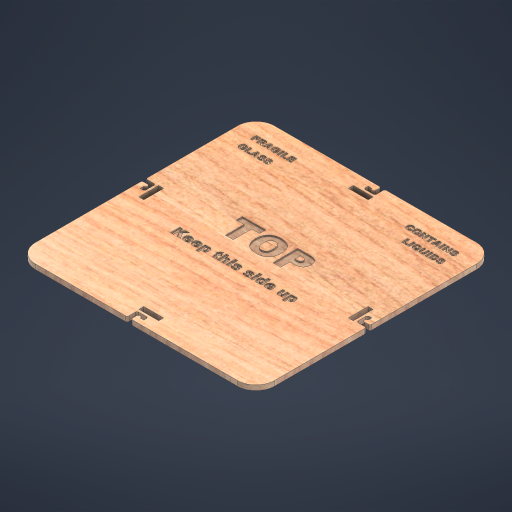
# Autodesk Inventor part: Lid
Saved by Autodesk Inventor 2024.1 (Build 281209000, 209)
## iProperties
Created: 2024-05-23
Part Number: Lid
Material: Wood (Birch)
Document SubType Name: Modeling
Designer: Tim Jäger
Density: 0.55 g/cm^3
Appearance: Birch - Natural Polished
Author: Tim Jäger
Autodesk Inventor part; units mm, degrees
(part 1 of 2)
ref_plane "YZ Plane" through (0, 0, 0) normal (1, 0, 0) x (0, 1, 0)
ref_plane "XZ Plane" through (0, 0, 0) normal (0, 1, 0) x (-1, 0, 0)
ref_plane "XY Plane" through (0, 0, 0) normal (0, 0, 1) x (1, 0, 0)
sketch "Sketch1" plane through (0, 0, 0) normal (0, 1, 0) x (-1, 0, 0)
  line L0 (-82, 97) -> (82, 97)
  line L1 (97, 82) -> (97, -82)
  line L2 (82, -97) -> (-82, -97)
  line L3 (-97, -82) -> (-97, 82)
  line L4 (-97, 97) -> (97, -97) construction
  line L5 (97, 97) -> (-97, -97) construction
  arc A0 (82, -97) -> (97, -82) centre (82, -82) ccw
  arc A1 (-97, -82) -> (-82, -97) centre (-82, -82) ccw
  arc A2 (-82, 97) -> (-97, 82) centre (-82, 82) ccw
  arc A3 (97, 82) -> (82, 97) centre (82, 82) ccw
  line L6 (97, -7.5) -> (89, -7.5)
  line L7 (89, -7.5) -> (89, 1.5)
  line L8 (89, 1.5) -> (91, 1.5)
  line L9 (91, 1.5) -> (91, -1.5) construction
  line L10 (91, -4.5) -> (97, -4.5)
  line L11 (91, 1.5) -> (92.5, 1.5)
  line L12 (92.5, 1.5) -> (92.5, -1.5)
  line L13 (92.5, -1.5) -> (91, -1.5)
  line L14 (91, -1.5) -> (91, 1.5) construction
  line L15 (91, -1.5) -> (91, -4.5)
  line L16 (-1.5, 89) -> (-1.5, 91)
  line L17 (-1.5, 91) -> (-1.5, 92.5)
  line L18 (-1.5, 91) -> (1.5, 91) construction
  line L19 (1.5, 91) -> (-1.5, 91) construction
  line L20 (-1.5, 92.5) -> (1.5, 92.5)
  line L21 (1.5, 91) -> (4.5, 91)
  line L22 (7.5, 89) -> (-1.5, 89)
  line L23 (4.5, 91) -> (4.5, 97)
  line L24 (7.5, 97) -> (7.5, 89)
  line L25 (1.5, 92.5) -> (1.5, 91)
  line L26 (-89, -1.5) -> (-91, -1.5)
  line L27 (-91, -1.5) -> (-92.5, -1.5)
  line L28 (-91, -1.5) -> (-91, 1.5) construction
  line L29 (-91, 1.5) -> (-91, -1.5) construction
  line L30 (-92.5, -1.5) -> (-92.5, 1.5)
  line L31 (-91, 1.5) -> (-91, 4.5)
  line L32 (-89, 7.5) -> (-89, -1.5)
  line L33 (-91, 4.5) -> (-97, 4.5)
  line L34 (-97, 7.5) -> (-89, 7.5)
  line L35 (-92.5, 1.5) -> (-91, 1.5)
  line L36 (1.5, -89) -> (1.5, -91)
  line L37 (1.5, -91) -> (1.5, -92.5)
  line L38 (1.5, -91) -> (-1.5, -91) construction
  line L39 (-1.5, -91) -> (1.5, -91) construction
  line L40 (1.5, -92.5) -> (-1.5, -92.5)
  line L41 (-1.5, -91) -> (-4.5, -91)
  line L42 (-7.5, -89) -> (1.5, -89)
  line L43 (-4.5, -91) -> (-4.5, -97)
  line L44 (-7.5, -97) -> (-7.5, -89)
  line L45 (-1.5, -92.5) -> (-1.5, -91)
  line L46 (8, -87) -> (-8, -87)
  line L47 (-8, -87) -> (-8, -83)
  line L48 (-8, -83) -> (8, -83)
  line L49 (8, -83) -> (8, -87)
  line L50 (87, -8) -> (83, -8)
  line L51 (83, -8) -> (83, 8)
  line L52 (83, 8) -> (87, 8)
  line L53 (87, 8) -> (87, -8)
  line L54 (8, 87) -> (8, 83)
  line L55 (8, 83) -> (-8, 83)
  line L56 (-8, 83) -> (-8, 87)
  line L57 (-8, 87) -> (8, 87)
  line L58 (-87, 8) -> (-83, 8)
  line L59 (-83, 8) -> (-83, -8)
  line L60 (-83, -8) -> (-87, -8)
  line L61 (-87, -8) -> (-87, 8)
  point P0 (0, 0)
  point P1 (93, -7.5)
  point P2 (92.5, 0)
  point P3 (0, 92.5)
  point P4 (7.5, 93)
  point P5 (-92.5, 0)
  point P6 (-93, 7.5)
  point P7 (0, -92.5)
  point P8 (-7.5, -93)
  point P9 (7.5, 97)
  point P10 (4.5, 97)
  point P11 (-97, 7.5)
  point P12 (-97, 4.5)
  point P13 (-7.5, -97)
  point P14 (-4.5, -97)
  point P15 (0, -87)
  point P16 (0, -83)
  point P17 (83, 0)
  point P18 (87, 0)
  point P19 (0, 0)
  point P20 (0, 83)
  point P21 (0, 87)
  point P22 (0, 0)
  point P23 (-83, 0)
  point P24 (-87, 0)
  point P25 (0, 0)
  dimension "d16" = 15
  dimension "d17" = 6
  dimension "d18" = 3
  dimension "d19" = 6
  dimension "d20" = 3
  dimension "d21" = 1.5
  dimension "d24" = 360
  dimension "d29" = 4
  dimension "d30" = 16
  dimension "d31" = 83
  dimension "d32" = 2
  dimension "d33" = 194
  dimension "d34" = 194
  dimension "d37" = 360
  constraints: 124 end point, 10 point on line, 8 perpendicular, 8 point on circle, 8 tangent, 6 midpoint, 6 parallel, 4 centre point, 4 horizontal, 3 equal radius, 2 coincident, 1 horizontal alignment, 1 vertical alignment, 128 other
  measures "d16" radius of A0
  measures "d17" distance between parallel lines of L1 L9
  measures "d18" distance from line of point (93, -7.5) L10
  measures "d19" distance of L8.end L10.start
  measures "d20" distance of L11.end L12.end
  measures "d21" distance of L12.end L9.end
  measures "d29" distance of L46.end L47.end
  measures "d30" distance of L46.start L46.end
  measures "d31" distance of point (0, 0) point (0, -83)
  measures "d32" distance between parallel lines of L7 L15
  measures "d33" distance between parallel lines of L1 L3
  measures "d34" distance between parallel lines of L0 L2
extrude "Extrusion1" add sketch "Sketch1" along normal blind 4 contours L0 L23 L21 L25 L20 L17 L16 L22 L24 A3 L1 L10 L15 L13 L12 L11 L8 L7 L6 A0 L2 L43 L41 L45 L40 L37 L36 L42 L44 A1 L3 L33 L31 L35 L30 L27 L26 L32 L34 A2
fillet "Fillet1" radius 1.5 24 edges at (-4.5, 2, 97) (-7.5, 2, 97) (-7.5, 2, 89) (-4.5, 2, 91) (1.5, 2, 89) (-1.5, 2, 91) (89, 2, 7.5) (97, 2, 7.5) (97, 2, 4.5) (91, 2, 4.5) (91, 2, 1.5) (89, 2, -1.5) (-1.5, 2, -89) (1.5, 2, -91) (4.5, 2, -91) (7.5, 2, -89) (4.5, 2, -97) (7.5, 2, -97) (-97, 2, -4.5) (-97, 2, -7.5) (-91, 2, -4.5) (-91, 2, -1.5) (-89, 2, 1.5) (-89, 2, -7.5)
sketch "Sketch2" plane through (0, 4, 0) normal (0, 1, 0) x (1, 0, 0)
  line L0 (-37.5, 25) -> (37.5, 25) construction
  line L1 (37.5, 25) -> (37.5, -5) construction
  line L2 (37.5, -5) -> (-37.5, -5) construction
  line L3 (-37.5, -5) -> (-37.5, 25) construction
  line L4 (-65, -10) -> (65, -10) construction
  line L5 (65, -10) -> (65, -25) construction
  line L6 (65, -25) -> (-65, -25) construction
  line L7 (-65, -25) -> (-65, -10) construction
  line L8 (0, 25) -> (0, -25) construction
  line L9 (-31.2031, 20.1697) -> (-12.3965, 20.1697)
  line L10 (-12.3965, 20.1697) -> (-12.3965, 15.2226)
  line L11 (-12.3965, 15.2226) -> (-18.7103, 15.2226)
  line L12 (-18.7103, 15.2226) -> (-18.7103, 0.1697)
  line L13 (-18.7103, 0.1697) -> (-24.8893, 0.1697)
  line L14 (-24.8893, 0.1697) -> (-24.8893, 15.2226)
  line L15 (-24.8893, 15.2226) -> (-31.2031, 15.2226)
  line L16 (-31.2031, 15.2226) -> (-31.2031, 20.1697)
  spline S0 degree 2 poles (-10.3754, 10.16) (-10.3754, 15.0493) (-4.9086, 20.5161) (-0.0385, 20.5161) knots 0 0 0 1 2 2 2
  spline S1 degree 2 poles (-0.0385, 20.5161) (4.9471, 20.5161) (10.3561, 15.1456) (10.3561, 10.314) knots 0 0 0 1 2 2 2
  spline S2 degree 2 poles (10.3561, 10.314) (10.3561, 6.8107) (7.9885, 2.3256) (3.5226, -0.1768) (0.1925, -0.1768) knots 0 0 0 1 2 3 3 3
  spline S3 degree 2 poles (0.1925, -0.1768) (-3.1761, -0.1768) (-7.6227, 1.9791) (-10.3754, 6.6567) (-10.3754, 10.16) knots 0 0 0 1 2 3 3 3
  spline S4 degree 2 poles (-4.1963, 10.1215) (-4.1963, 7.0994) (-1.9442, 4.443) (0, 4.443) knots 0 0 0 1 2 2 2
  spline S5 degree 2 poles (0, 4.443) (1.9827, 4.443) (4.1771, 7.0416) (4.1771, 10.391) knots 0 0 0 1 2 2 2
  spline S6 degree 2 poles (4.1771, 10.391) (4.1771, 13.2207) (1.9057, 15.8386) (-0.0577, 15.8386) knots 0 0 0 1 2 2 2
  spline S7 degree 2 poles (-0.0577, 15.8386) (-1.9249, 15.8386) (-4.1963, 13.1822) (-4.1963, 10.1215) knots 0 0 0 1 2 2 2
  line L17 (13.667, 20.1697) -> (23.9461, 20.1697)
  spline S8 degree 2 poles (23.9461, 20.1697) (27.2955, 20.1697) (30.6449, 16.9743) (30.6449, 14.0291) knots 0 0 0 1 2 2 2
  spline S9 degree 2 poles (30.6449, 14.0291) (30.6449, 10.9878) (27.0067, 7.5806) (23.2724, 7.5806) knots 0 0 0 1 2 2 2
  line L18 (23.2724, 7.5806) -> (19.8845, 7.5806)
  line L19 (19.8845, 7.5806) -> (19.8845, 0.1697)
  line L20 (19.8845, 0.1697) -> (13.667, 0.1697)
  line L21 (13.667, 0.1697) -> (13.667, 20.1697)
  line L22 (19.8845, 11.6422) -> (21.3859, 11.6422)
  spline S10 degree 2 poles (21.3859, 11.6422) (23.1761, 11.6422) (24.6198, 12.8934) (24.6198, 13.8559) knots 0 0 0 1 2 2 2
  spline S11 degree 2 poles (24.6198, 13.8559) (24.6198, 14.7991) (23.3686, 16.1081) (21.6362, 16.1081) knots 0 0 0 1 2 2 2
  line L23 (21.6362, 16.1081) -> (19.8845, 16.1081)
  line L24 (19.8845, 16.1081) -> (19.8845, 11.6422)
  line L25 (-49.0315, -12.7178) -> (-46.7144, -12.7178)
  line L26 (-46.7144, -12.7178) -> (-46.7144, -15.5546)
  line L27 (-46.7144, -15.5546) -> (-44.2818, -12.7178)
  line L28 (-44.2818, -12.7178) -> (-41.1995, -12.7178)
  line L29 (-41.1995, -12.7178) -> (-43.9353, -15.5474)
  line L30 (-43.9353, -15.5474) -> (-41.0768, -20.2178)
  line L31 (-41.0768, -20.2178) -> (-43.9353, -20.2178)
  line L32 (-43.9353, -20.2178) -> (-45.5161, -17.1355)
  line L33 (-45.5161, -17.1355) -> (-46.7144, -18.3987)
  line L34 (-46.7144, -18.3987) -> (-46.7144, -20.2178)
  line L35 (-46.7144, -20.2178) -> (-49.0315, -20.2178)
  line L36 (-49.0315, -20.2178) -> (-49.0315, -12.7178)
  line L37 (-34.4141, -18.0161) -> (-38.5864, -18.0161)
  spline S12 degree 2 poles (-38.5864, -18.0161) (-38.5286, -18.5214) (-38.3121, -18.7668) knots 0 0 0 1 1 1
  spline S13 degree 2 poles (-38.3121, -18.7668) (-38.0161, -19.1205) (-37.5253, -19.1205) knots 0 0 0 1 1 1
  spline S14 degree 2 poles (-37.5253, -19.1205) (-37.2221, -19.1205) (-36.9406, -18.969) knots 0 0 0 1 1 1
  spline S15 degree 2 poles (-36.9406, -18.969) (-36.7745, -18.8679) (-36.5796, -18.6225) knots 0 0 0 1 1 1
  line L38 (-36.5796, -18.6225) -> (-34.5296, -18.8102)
  spline S16 degree 2 poles (-34.5296, -18.8102) (-34.9988, -19.6258) (-36.3342, -20.3405) (-37.5758, -20.3405) knots 0 0 0 1 2 2 2
  spline S17 degree 2 poles (-37.5758, -20.3405) (-38.6586, -20.3405) (-39.8929, -19.7341) (-40.7086, -18.4059) (-40.7086, -17.5108) knots 0 0 0 1 2 3 3 3
  spline S18 degree 2 poles (-40.7086, -17.5108) (-40.7086, -16.2332) (-39.0772, -14.6595) (-37.6408, -14.6595) knots 0 0 0 1 2 2 2
  spline S19 degree 2 poles (-37.6408, -14.6595) (-36.4714, -14.6595) (-35.1215, -15.3669) (-34.4141, -16.7096) (-34.4141, -17.7779) knots 0 0 0 1 2 3 3 3
  line L39 (-34.4141, -17.7779) -> (-34.4141, -18.0161)
  spline S20 degree 2 poles (-36.5363, -17.02) (-36.5941, -16.4136) (-37.121, -15.8939) (-37.5541, -15.8939) knots 0 0 0 1 2 2 2
  spline S21 degree 2 poles (-37.5541, -15.8939) (-38.045, -15.8939) (-38.341, -16.2909) knots 0 0 0 1 1 1
  spline S22 degree 2 poles (-38.341, -16.2909) (-38.5286, -16.5363) (-38.5792, -17.02) knots 0 0 0 1 1 1
  line L40 (-38.5792, -17.02) -> (-36.5363, -17.02)
  line L41 (-27.4194, -18.0161) -> (-31.5917, -18.0161)
  spline S23 degree 2 poles (-31.5917, -18.0161) (-31.5339, -18.5214) (-31.3174, -18.7668) knots 0 0 0 1 1 1
  spline S24 degree 2 poles (-31.3174, -18.7668) (-31.0214, -19.1205) (-30.5306, -19.1205) knots 0 0 0 1 1 1
  spline S25 degree 2 poles (-30.5306, -19.1205) (-30.2274, -19.1205) (-29.9459, -18.969) knots 0 0 0 1 1 1
  spline S26 degree 2 poles (-29.9459, -18.969) (-29.7798, -18.8679) (-29.5849, -18.6225) knots 0 0 0 1 1 1
  line L42 (-29.5849, -18.6225) -> (-27.5349, -18.8102)
  spline S27 degree 2 poles (-27.5349, -18.8102) (-28.0041, -19.6258) (-29.3395, -20.3405) (-30.5811, -20.3405) knots 0 0 0 1 2 2 2
  spline S28 degree 2 poles (-30.5811, -20.3405) (-31.6639, -20.3405) (-32.8982, -19.7341) (-33.7139, -18.4059) (-33.7139, -17.5108) knots 0 0 0 1 2 3 3 3
  spline S29 degree 2 poles (-33.7139, -17.5108) (-33.7139, -16.2332) (-32.0825, -14.6595) (-30.6461, -14.6595) knots 0 0 0 1 2 2 2
  spline S30 degree 2 poles (-30.6461, -14.6595) (-29.4767, -14.6595) (-28.1268, -15.3669) (-27.4194, -16.7096) (-27.4194, -17.7779) knots 0 0 0 1 2 3 3 3
  line L43 (-27.4194, -17.7779) -> (-27.4194, -18.0161)
  spline S31 degree 2 poles (-29.5416, -17.02) (-29.5994, -16.4136) (-30.1263, -15.8939) (-30.5594, -15.8939) knots 0 0 0 1 2 2 2
  spline S32 degree 2 poles (-30.5594, -15.8939) (-31.0503, -15.8939) (-31.3462, -16.2909) knots 0 0 0 1 1 1
  spline S33 degree 2 poles (-31.3462, -16.2909) (-31.5339, -16.5363) (-31.5845, -17.02) knots 0 0 0 1 1 1
  line L44 (-31.5845, -17.02) -> (-29.5416, -17.02)
  line L45 (-26.4449, -22.2822) -> (-26.4449, -14.7822)
  line L46 (-26.4449, -14.7822) -> (-24.4959, -14.7822)
  line L47 (-24.4959, -14.7822) -> (-24.4959, -15.5835)
  spline S34 degree 2 poles (-24.4959, -15.5835) (-24.0917, -15.0782) (-23.7596, -14.8977) knots 0 0 0 1 1 1
  spline S35 degree 2 poles (-23.7596, -14.8977) (-23.2976, -14.6595) (-22.749, -14.6595) knots 0 0 0 1 1 1
  spline S36 degree 2 poles (-22.749, -14.6595) (-21.659, -14.6595) (-20.468, -16.327) (-20.468, -17.5541) knots 0 0 0 1 2 2 2
  spline S37 degree 2 poles (-20.468, -17.5541) (-20.468, -18.9112) (-21.7673, -20.3405) (-22.7563, -20.3405) knots 0 0 0 1 2 2 2
  spline S38 degree 2 poles (-22.7563, -20.3405) (-23.2399, -20.3405) (-24.0339, -20.0156) (-24.3443, -19.6908) knots 0 0 0 1 2 2 2
  line L48 (-24.3443, -19.6908) -> (-24.3443, -22.2822)
  line L49 (-24.3443, -22.2822) -> (-26.4449, -22.2822)
  spline S39 degree 2 poles (-24.3588, -17.5108) (-24.3588, -18.1605) (-23.8174, -18.7813) (-23.4059, -18.7813) knots 0 0 0 1 2 2 2
  spline S40 degree 2 poles (-23.4059, -18.7813) (-23.045, -18.7813) (-22.5541, -18.1821) (-22.5541, -17.4675) knots 0 0 0 1 2 2 2
  spline S41 degree 2 poles (-22.5541, -17.4675) (-22.5541, -16.8106) (-23.0666, -16.1898) (-23.4348, -16.1898) knots 0 0 0 1 2 2 2
  spline S42 degree 2 poles (-23.4348, -16.1898) (-23.8318, -16.1898) (-24.3588, -16.8106) (-24.3588, -17.5108) knots 0 0 0 1 2 2 2
  line L50 (-13.4589, -12.7178) -> (-13.4589, -14.7822)
  line L51 (-13.4589, -14.7822) -> (-12.3111, -14.7822)
  line L52 (-12.3111, -14.7822) -> (-12.3111, -16.3053)
  line L53 (-12.3111, -16.3053) -> (-13.4589, -16.3053)
  line L54 (-13.4589, -16.3053) -> (-13.4589, -18.2327)
  spline S43 degree 2 poles (-13.4589, -18.2327) (-13.4589, -18.5792) (-13.3939, -18.6947) knots 0 0 0 1 1 1
  spline S44 degree 2 poles (-13.3939, -18.6947) (-13.2928, -18.8679) (-13.033, -18.8679) knots 0 0 0 1 1 1
  spline S45 degree 2 poles (-13.033, -18.8679) (-12.802, -18.8679) (-12.3905, -18.738) knots 0 0 0 1 1 1
  line L55 (-12.3905, -18.738) -> (-12.2389, -20.1744)
  spline S46 degree 2 poles (-12.2389, -20.1744) (-13.0113, -20.3405) (-13.6826, -20.3405) knots 0 0 0 1 1 1
  spline S47 degree 2 poles (-13.6826, -20.3405) (-14.455, -20.3405) (-15.1913, -19.9435) (-15.545, -19.1278) (-15.545, -18.2182) knots 0 0 0 1 2 3 3 3
  line L56 (-15.545, -18.2182) -> (-15.545, -16.3053)
  line L57 (-15.545, -16.3053) -> (-16.3102, -16.3053)
  line L58 (-16.3102, -16.3053) -> (-16.3102, -14.7822)
  line L59 (-16.3102, -14.7822) -> (-15.545, -14.7822)
  line L60 (-15.545, -14.7822) -> (-15.545, -13.7861)
  line L61 (-15.545, -13.7861) -> (-13.4589, -12.7178)
  line L62 (-11.315, -12.7178) -> (-9.2288, -12.7178)
  line L63 (-9.2288, -12.7178) -> (-9.2288, -15.4752)
  spline S48 degree 2 poles (-9.2288, -15.4752) (-8.8029, -15.0349) (-7.9656, -14.6595) (-7.3953, -14.6595) knots 0 0 0 1 2 2 2
  spline S49 degree 2 poles (-7.3953, -14.6595) (-6.5436, -14.6595) (-5.5691, -15.6918) (-5.5691, -16.7601) knots 0 0 0 1 2 2 2
  line L64 (-5.5691, -16.7601) -> (-5.5691, -20.2178)
  line L65 (-5.5691, -20.2178) -> (-7.6624, -20.2178)
  line L66 (-7.6624, -20.2178) -> (-7.6624, -17.2293)
  spline S50 degree 2 poles (-7.6624, -17.2293) (-7.6624, -16.7168) (-8.0378, -16.2909) (-8.3843, -16.2909) knots 0 0 0 1 2 2 2
  spline S51 degree 2 poles (-8.3843, -16.2909) (-8.7596, -16.2909) (-9.2288, -16.8612) (-9.2288, -17.6047) knots 0 0 0 1 2 2 2
  line L67 (-9.2288, -17.6047) -> (-9.2288, -20.2178)
  line L68 (-9.2288, -20.2178) -> (-11.315, -20.2178)
  line L69 (-11.315, -20.2178) -> (-11.315, -12.7178)
  line L70 (-4.2409, -14.7822) -> (-2.1547, -14.7822)
  line L71 (-2.1547, -14.7822) -> (-2.1547, -20.2178)
  line L72 (-2.1547, -20.2178) -> (-4.2409, -20.2178)
  line L73 (-4.2409, -20.2178) -> (-4.2409, -14.7822)
  line L74 (-4.2409, -12.7178) -> (-2.1547, -12.7178)
  line L75 (-2.1547, -12.7178) -> (-2.1547, -14.1326)
  line L76 (-2.1547, -14.1326) -> (-4.2409, -14.1326)
  line L77 (-4.2409, -14.1326) -> (-4.2409, -12.7178)
  line L78 (-1.1947, -18.7091) -> (0.8698, -18.5142)
  spline S52 degree 2 poles (0.8698, -18.5142) (0.9998, -18.8823) (1.4617, -19.2) (1.8443, -19.2) knots 0 0 0 1 2 2 2
  spline S53 degree 2 poles (1.8443, -19.2) (2.2702, -19.2) (2.5012, -19.0195) knots 0 0 0 1 1 1
  spline S54 degree 2 poles (2.5012, -19.0195) (2.6817, -18.8896) (2.6817, -18.6874) knots 0 0 0 1 1 1
  spline S55 degree 2 poles (2.6817, -18.6874) (2.6817, -18.4637) (2.4435, -18.341) knots 0 0 0 1 1 1
  spline S56 degree 2 poles (2.4435, -18.341) (2.2702, -18.2543) (1.5484, -18.1244) knots 0 0 0 1 1 1
  spline S57 degree 2 poles (1.5484, -18.1244) (0.4584, -17.9367) (-0.3862, -17.6119) (-0.9637, -16.8467) (-0.9637, -16.3559) knots 0 0 0 1 2 3 3 3
  spline S58 degree 2 poles (-0.9637, -16.3559) (-0.9637, -15.8217) (-0.3357, -15.0421) (0.7543, -14.6595) (1.6783, -14.6595) knots 0 0 0 1 2 3 3 3
  spline S59 degree 2 poles (1.6783, -14.6595) (2.6528, -14.6595) (3.5768, -14.9555) (4.1975, -15.5763) (4.3997, -16.1104) knots 0 0 0 1 2 3 3 3
  line L79 (4.3997, -16.1104) -> (2.4218, -16.3053)
  spline S60 degree 2 poles (2.4218, -16.3053) (2.3424, -16.0455) (2.1692, -15.9228) knots 0 0 0 1 1 1
  spline S61 degree 2 poles (2.1692, -15.9228) (1.9237, -15.7567) (1.57, -15.7567) knots 0 0 0 1 1 1
  spline S62 degree 2 poles (1.57, -15.7567) (1.2235, -15.7567) (0.8987, -16.0094) (0.8987, -16.1898) knots 0 0 0 1 2 2 2
  spline S63 degree 2 poles (0.8987, -16.1898) (0.8987, -16.3847) (1.108, -16.4858) knots 0 0 0 1 1 1
  spline S64 degree 2 poles (1.108, -16.4858) (1.3102, -16.5941) (1.9959, -16.6735) knots 0 0 0 1 1 1
  spline S65 degree 2 poles (1.9959, -16.6735) (3.0354, -16.789) (4.0532, -17.2077) (4.5873, -17.9872) (4.5873, -18.4492) knots 0 0 0 1 2 3 3 3
  spline S66 degree 2 poles (4.5873, -18.4492) (4.5873, -18.9256) (4.0171, -19.8135) (2.7972, -20.3405) (1.7433, -20.3405) knots 0 0 0 1 2 3 3 3
  spline S67 degree 2 poles (1.7433, -20.3405) (0.249, -20.3405) (-1.0142, -19.4887) (-1.1947, -18.7091) knots 0 0 0 1 2 2 2
  line L80 (8.7019, -18.7091) -> (10.7664, -18.5142)
  spline S68 degree 2 poles (10.7664, -18.5142) (10.8963, -18.8823) (11.3583, -19.2) (11.7409, -19.2) knots 0 0 0 1 2 2 2
  spline S69 degree 2 poles (11.7409, -19.2) (12.1667, -19.2) (12.3977, -19.0195) knots 0 0 0 1 1 1
  spline S70 degree 2 poles (12.3977, -19.0195) (12.5782, -18.8896) (12.5782, -18.6874) knots 0 0 0 1 1 1
  spline S71 degree 2 poles (12.5782, -18.6874) (12.5782, -18.4637) (12.34, -18.341) knots 0 0 0 1 1 1
  spline S72 degree 2 poles (12.34, -18.341) (12.1667, -18.2543) (11.4449, -18.1244) knots 0 0 0 1 1 1
  spline S73 degree 2 poles (11.4449, -18.1244) (10.3549, -17.9367) (9.5103, -17.6119) (8.9329, -16.8467) (8.9329, -16.3559) knots 0 0 0 1 2 3 3 3
  spline S74 degree 2 poles (8.9329, -16.3559) (8.9329, -15.8217) (9.5609, -15.0421) (10.6509, -14.6595) (11.5748, -14.6595) knots 0 0 0 1 2 3 3 3
  spline S75 degree 2 poles (11.5748, -14.6595) (12.5493, -14.6595) (13.4733, -14.9555) (14.0941, -15.5763) (14.2962, -16.1104) knots 0 0 0 1 2 3 3 3
  line L81 (14.2962, -16.1104) -> (12.3183, -16.3053)
  spline S76 degree 2 poles (12.3183, -16.3053) (12.2389, -16.0455) (12.0657, -15.9228) knots 0 0 0 1 1 1
  spline S77 degree 2 poles (12.0657, -15.9228) (11.8203, -15.7567) (11.4666, -15.7567) knots 0 0 0 1 1 1
  spline S78 degree 2 poles (11.4666, -15.7567) (11.1201, -15.7567) (10.7952, -16.0094) (10.7952, -16.1898) knots 0 0 0 1 2 2 2
  spline S79 degree 2 poles (10.7952, -16.1898) (10.7952, -16.3847) (11.0046, -16.4858) knots 0 0 0 1 1 1
  spline S80 degree 2 poles (11.0046, -16.4858) (11.2067, -16.5941) (11.8924, -16.6735) knots 0 0 0 1 1 1
  spline S81 degree 2 poles (11.8924, -16.6735) (12.9319, -16.789) (13.9497, -17.2077) (14.4839, -17.9872) (14.4839, -18.4492) knots 0 0 0 1 2 3 3 3
  spline S82 degree 2 poles (14.4839, -18.4492) (14.4839, -18.9256) (13.9136, -19.8135) (12.6937, -20.3405) (11.6398, -20.3405) knots 0 0 0 1 2 3 3 3
  spline S83 degree 2 poles (11.6398, -20.3405) (10.1456, -20.3405) (8.8823, -19.4887) (8.7019, -18.7091) knots 0 0 0 1 2 2 2
  line L82 (15.5522, -14.7822) -> (17.6384, -14.7822)
  line L83 (17.6384, -14.7822) -> (17.6384, -20.2178)
  line L84 (17.6384, -20.2178) -> (15.5522, -20.2178)
  line L85 (15.5522, -20.2178) -> (15.5522, -14.7822)
  line L86 (15.5522, -12.7178) -> (17.6384, -12.7178)
  line L87 (17.6384, -12.7178) -> (17.6384, -14.1326)
  line L88 (17.6384, -14.1326) -> (15.5522, -14.1326)
  line L89 (15.5522, -14.1326) -> (15.5522, -12.7178)
  line L90 (24.6836, -12.7178) -> (24.6836, -20.2178)
  line L91 (24.6836, -20.2178) -> (22.7346, -20.2178)
  line L92 (22.7346, -20.2178) -> (22.7346, -19.4165)
  spline S84 degree 2 poles (22.7346, -19.4165) (22.3304, -19.929) (21.9911, -20.1023) knots 0 0 0 1 1 1
  spline S85 degree 2 poles (21.9911, -20.1023) (21.5363, -20.3405) (20.9877, -20.3405) knots 0 0 0 1 1 1
  spline S86 degree 2 poles (20.9877, -20.3405) (19.8761, -20.3405) (18.7067, -18.6513) (18.7067, -17.4459) knots 0 0 0 1 2 2 2
  spline S87 degree 2 poles (18.7067, -17.4459) (18.7067, -16.096) (19.9988, -14.6595) (20.9949, -14.6595) knots 0 0 0 1 2 2 2
  spline S88 degree 2 poles (20.9949, -14.6595) (21.4858, -14.6595) (22.2798, -14.9844) (22.583, -15.3164) knots 0 0 0 1 2 2 2
  line L93 (22.583, -15.3164) -> (22.583, -12.7178)
  line L94 (22.583, -12.7178) -> (24.6836, -12.7178)
  spline S89 degree 2 poles (22.5975, -17.4892) (22.5975, -16.8467) (22.0561, -16.2187) (21.6446, -16.2187) knots 0 0 0 1 2 2 2
  spline S90 degree 2 poles (21.6446, -16.2187) (21.2837, -16.2187) (20.7928, -16.8251) (20.7928, -17.5325) knots 0 0 0 1 2 2 2
  spline S91 degree 2 poles (20.7928, -17.5325) (20.7928, -18.1966) (21.2981, -18.8174) (21.6735, -18.8174) knots 0 0 0 1 2 2 2
  spline S92 degree 2 poles (21.6735, -18.8174) (22.0705, -18.8174) (22.5975, -18.1966) (22.5975, -17.4892) knots 0 0 0 1 2 2 2
  line L95 (31.9959, -18.0161) -> (27.8236, -18.0161)
  spline S93 degree 2 poles (27.8236, -18.0161) (27.8814, -18.5214) (28.0979, -18.7668) knots 0 0 0 1 1 1
  spline S94 degree 2 poles (28.0979, -18.7668) (28.3939, -19.1205) (28.8847, -19.1205) knots 0 0 0 1 1 1
  spline S95 degree 2 poles (28.8847, -19.1205) (29.1879, -19.1205) (29.4694, -18.969) knots 0 0 0 1 1 1
  spline S96 degree 2 poles (29.4694, -18.969) (29.6355, -18.8679) (29.8304, -18.6225) knots 0 0 0 1 1 1
  line L96 (29.8304, -18.6225) -> (31.8804, -18.8102)
  spline S97 degree 2 poles (31.8804, -18.8102) (31.4112, -19.6258) (30.0758, -20.3405) (28.8342, -20.3405) knots 0 0 0 1 2 2 2
  spline S98 degree 2 poles (28.8342, -20.3405) (27.7514, -20.3405) (26.5171, -19.7341) (25.7014, -18.4059) (25.7014, -17.5108) knots 0 0 0 1 2 3 3 3
  spline S99 degree 2 poles (25.7014, -17.5108) (25.7014, -16.2332) (27.3328, -14.6595) (28.7693, -14.6595) knots 0 0 0 1 2 2 2
  spline S100 degree 2 poles (28.7693, -14.6595) (29.9386, -14.6595) (31.2885, -15.3669) (31.9959, -16.7096) (31.9959, -17.7779) knots 0 0 0 1 2 3 3 3
  line L97 (31.9959, -17.7779) -> (31.9959, -18.0161)
  spline S101 degree 2 poles (29.8737, -17.02) (29.8159, -16.4136) (29.289, -15.8939) (28.8559, -15.8939) knots 0 0 0 1 2 2 2
  spline S102 degree 2 poles (28.8559, -15.8939) (28.365, -15.8939) (28.0691, -16.2909) knots 0 0 0 1 1 1
  spline S103 degree 2 poles (28.0691, -16.2909) (27.8814, -16.5363) (27.8308, -17.02) knots 0 0 0 1 1 1
  line L98 (27.8308, -17.02) -> (29.8737, -17.02)
  line L99 (42.174, -20.2178) -> (40.225, -20.2178)
  line L100 (40.225, -20.2178) -> (40.225, -19.3371)
  spline S104 degree 2 poles (40.225, -19.3371) (39.7919, -19.8785) (38.904, -20.3405) (38.2616, -20.3405) knots 0 0 0 1 2 2 2
  spline S105 degree 2 poles (38.2616, -20.3405) (37.4026, -20.3405) (36.4281, -19.3082) (36.4281, -18.2399) knots 0 0 0 1 2 2 2
  line L101 (36.4281, -18.2399) -> (36.4281, -14.7822)
  line L102 (36.4281, -14.7822) -> (38.5214, -14.7822)
  line L103 (38.5214, -14.7822) -> (38.5214, -17.7707)
  spline S106 degree 2 poles (38.5214, -17.7707) (38.5214, -18.2832) (38.8968, -18.7163) (39.2433, -18.7163) knots 0 0 0 1 2 2 2
  spline S107 degree 2 poles (39.2433, -18.7163) (39.6114, -18.7163) (40.0878, -18.1461) (40.0878, -17.4026) knots 0 0 0 1 2 2 2
  line L104 (40.0878, -17.4026) -> (40.0878, -14.7822)
  line L105 (40.0878, -14.7822) -> (42.174, -14.7822)
  line L106 (42.174, -14.7822) -> (42.174, -20.2178)
  line L107 (43.4589, -22.2822) -> (43.4589, -14.7822)
  line L108 (43.4589, -14.7822) -> (45.4078, -14.7822)
  line L109 (45.4078, -14.7822) -> (45.4078, -15.5835)
  spline S108 degree 2 poles (45.4078, -15.5835) (45.8121, -15.0782) (46.1441, -14.8977) knots 0 0 0 1 1 1
  spline S109 degree 2 poles (46.1441, -14.8977) (46.6061, -14.6595) (47.1547, -14.6595) knots 0 0 0 1 1 1
  spline S110 degree 2 poles (47.1547, -14.6595) (48.2447, -14.6595) (49.4358, -16.327) (49.4358, -17.5541) knots 0 0 0 1 2 2 2
  spline S111 degree 2 poles (49.4358, -17.5541) (49.4358, -18.9112) (48.1364, -20.3405) (47.1475, -20.3405) knots 0 0 0 1 2 2 2
  spline S112 degree 2 poles (47.1475, -20.3405) (46.6639, -20.3405) (45.8698, -20.0156) (45.5594, -19.6908) knots 0 0 0 1 2 2 2
  line L110 (45.5594, -19.6908) -> (45.5594, -22.2822)
  line L111 (45.5594, -22.2822) -> (43.4589, -22.2822)
  spline S113 degree 2 poles (45.545, -17.5108) (45.545, -18.1605) (46.0864, -18.7813) (46.4978, -18.7813) knots 0 0 0 1 2 2 2
  spline S114 degree 2 poles (46.4978, -18.7813) (46.8588, -18.7813) (47.3496, -18.1821) (47.3496, -17.4675) knots 0 0 0 1 2 2 2
  spline S115 degree 2 poles (47.3496, -17.4675) (47.3496, -16.8106) (46.8371, -16.1898) (46.469, -16.1898) knots 0 0 0 1 2 2 2
  spline S116 degree 2 poles (46.469, -16.1898) (46.0719, -16.1898) (45.545, -16.8106) (45.545, -17.5108) knots 0 0 0 1 2 2 2
  point P0 (0, 0)
  point P1 (37.5, 10)
  point P2 (41.0562, -38.1947)
  point P3 (6.8053, -25.8381)
  point P4 (65, -17.5)
  point P5 (0, -10)
  point P6 (0, 0)
  dimension "d39" = 15
  dimension "d40" = 130
  dimension "d41" = 75
  dimension "d42" = 30
  dimension "d43" = 5
  constraints: 6 midpoint, 2 end point, 2 vertical alignment, 1 coincident, 1 vertical, 4 other
  measures "d39" distance of L4.end L5.end
  measures "d40" distance of L7.end L4.end
  measures "d41" distance of L1.end L2.end
  measures "d42" distance of L0.end L1.end
  measures "d43" distance between parallel lines of L4 L2
extrude "Extrusion2" cut sketch "Sketch2" against normal blind 1
sketch "Sketch3" plane through (0, 4, 0) normal (0, 1, 0) x (1, 0, 0)
  line L0 (-83, 83) -> (-43, 83) construction
  line L1 (-43, 83) -> (-43, 63) construction
  line L2 (-43, 63) -> (-83, 63) construction
  line L3 (-83, 63) -> (-83, 83) construction
  line L4 (38, 83) -> (83, 83) construction
  line L5 (83, 83) -> (83, 63) construction
  line L6 (83, 63) -> (38, 63) construction
  line L7 (38, 63) -> (38, 83) construction
  line L8 (45.6805, 79.9586) -> (47.0327, 79.5496)
  spline S0 degree 2 poles (47.0327, 79.5496) (46.898, 78.9817) (46.3109, 78.2166) (45.4398, 77.8268) (44.7709, 77.8268) knots 0 0 0 1 2 3 3 3
  spline S1 degree 2 poles (44.7709, 77.8268) (43.9528, 77.8268) (42.923, 78.3032) (42.1723, 79.4966) (42.1723, 80.4254) knots 0 0 0 1 2 3 3 3
  spline S2 degree 2 poles (42.1723, 80.4254) (42.1723, 81.667) (43.4909, 83) (44.6987, 83) knots 0 0 0 1 2 2 2
  spline S3 degree 2 poles (44.6987, 83) (45.642, 83) (46.7199, 82.2348) (46.9846, 81.4456) knots 0 0 0 1 2 2 2
  line L9 (46.9846, 81.4456) -> (45.6179, 81.1424)
  spline S4 degree 2 poles (45.6179, 81.1424) (45.5457, 81.3686) (45.4687, 81.4745) knots 0 0 0 1 1 1
  spline S5 degree 2 poles (45.4687, 81.4745) (45.3388, 81.6526) (44.9634, 81.845) (44.7324, 81.845) knots 0 0 0 1 2 2 2
  spline S6 degree 2 poles (44.7324, 81.845) (44.2127, 81.845) (43.9336, 81.4216) knots 0 0 0 1 1 1
  spline S7 degree 2 poles (43.9336, 81.4216) (43.7218, 81.1088) (43.7218, 80.435) knots 0 0 0 1 1 1
  spline S8 degree 2 poles (43.7218, 80.435) (43.7218, 79.6025) (44.2271, 78.9865) (44.6843, 78.9865) knots 0 0 0 1 2 2 2
  spline S9 degree 2 poles (44.6843, 78.9865) (45.127, 78.9865) (45.5794, 79.4822) (45.6805, 79.9586) knots 0 0 0 1 2 2 2
  spline S10 degree 2 poles (47.5958, 80.411) (47.5958, 81.6333) (48.9625, 83) (50.18, 83) knots 0 0 0 1 2 2 2
  spline S11 degree 2 poles (50.18, 83) (51.4264, 83) (52.7786, 81.6574) (52.7786, 80.4495) knots 0 0 0 1 2 2 2
  spline S12 degree 2 poles (52.7786, 80.4495) (52.7786, 79.5736) (52.1867, 78.4524) (51.0703, 77.8268) (50.2377, 77.8268) knots 0 0 0 1 2 3 3 3
  spline S13 degree 2 poles (50.2377, 77.8268) (49.3956, 77.8268) (48.2839, 78.3657) (47.5958, 79.5351) (47.5958, 80.411) knots 0 0 0 1 2 3 3 3
  spline S14 degree 2 poles (49.1405, 80.4013) (49.1405, 79.6458) (49.7036, 78.9817) (50.1896, 78.9817) knots 0 0 0 1 2 2 2
  spline S15 degree 2 poles (50.1896, 78.9817) (50.6853, 78.9817) (51.2339, 79.6314) (51.2339, 80.4687) knots 0 0 0 1 2 2 2
  spline S16 degree 2 poles (51.2339, 80.4687) (51.2339, 81.1761) (50.666, 81.8306) (50.1752, 81.8306) knots 0 0 0 1 2 2 2
  spline S17 degree 2 poles (50.1752, 81.8306) (49.7084, 81.8306) (49.1405, 81.1665) (49.1405, 80.4013) knots 0 0 0 1 2 2 2
  line L10 (53.6208, 82.9134) -> (55.0645, 82.9134)
  line L11 (55.0645, 82.9134) -> (56.9509, 80.1463)
  line L12 (56.9509, 80.1463) -> (56.9509, 82.9134)
  line L13 (56.9509, 82.9134) -> (58.409, 82.9134)
  line L14 (58.409, 82.9134) -> (58.409, 77.9134)
  line L15 (58.409, 77.9134) -> (56.9509, 77.9134)
  line L16 (56.9509, 77.9134) -> (55.0741, 80.666)
  line L17 (55.0741, 80.666) -> (55.0741, 77.9134)
  line L18 (55.0741, 77.9134) -> (53.6208, 77.9134)
  line L19 (53.6208, 77.9134) -> (53.6208, 82.9134)
  line L20 (59.0828, 82.9134) -> (63.7844, 82.9134)
  line L21 (63.7844, 82.9134) -> (63.7844, 81.6766)
  line L22 (63.7844, 81.6766) -> (62.206, 81.6766)
  line L23 (62.206, 81.6766) -> (62.206, 77.9134)
  line L24 (62.206, 77.9134) -> (60.6612, 77.9134)
  line L25 (60.6612, 77.9134) -> (60.6612, 81.6766)
  line L26 (60.6612, 81.6766) -> (59.0828, 81.6766)
  line L27 (59.0828, 81.6766) -> (59.0828, 82.9134)
  line L28 (67.5573, 78.7411) -> (65.8008, 78.7411)
  line L29 (65.8008, 78.7411) -> (65.5553, 77.9134)
  line L30 (65.5553, 77.9134) -> (63.9769, 77.9134)
  line L31 (63.9769, 77.9134) -> (65.8585, 82.9134)
  line L32 (65.8585, 82.9134) -> (67.5476, 82.9134)
  line L33 (67.5476, 82.9134) -> (69.4244, 77.9134)
  line L34 (69.4244, 77.9134) -> (67.8075, 77.9134)
  line L35 (67.8075, 77.9134) -> (67.5573, 78.7411)
  line L36 (67.2348, 79.8239) -> (66.6862, 81.6189)
  line L37 (66.6862, 81.6189) -> (66.1376, 79.8239)
  line L38 (66.1376, 79.8239) -> (67.2348, 79.8239)
  line L39 (69.9827, 82.9134) -> (71.5322, 82.9134)
  line L40 (71.5322, 82.9134) -> (71.5322, 77.9134)
  line L41 (71.5322, 77.9134) -> (69.9827, 77.9134)
  line L42 (69.9827, 77.9134) -> (69.9827, 82.9134)
  line L43 (72.6487, 82.9134) -> (74.0924, 82.9134)
  line L44 (74.0924, 82.9134) -> (75.9788, 80.1463)
  line L45 (75.9788, 80.1463) -> (75.9788, 82.9134)
  line L46 (75.9788, 82.9134) -> (77.437, 82.9134)
  line L47 (77.437, 82.9134) -> (77.437, 77.9134)
  line L48 (77.437, 77.9134) -> (75.9788, 77.9134)
  line L49 (75.9788, 77.9134) -> (74.102, 80.666)
  line L50 (74.102, 80.666) -> (74.102, 77.9134)
  line L51 (74.102, 77.9134) -> (72.6487, 77.9134)
  line L52 (72.6487, 77.9134) -> (72.6487, 82.9134)
  line L53 (78.1925, 79.5688) -> (79.6651, 79.6603)
  spline S18 degree 2 poles (79.6651, 79.6603) (79.7132, 79.2993) (79.8576, 79.1116) knots 0 0 0 1 1 1
  spline S19 degree 2 poles (79.8576, 79.1116) (80.0982, 78.8085) (80.5457, 78.8085) knots 0 0 0 1 1 1
  spline S20 degree 2 poles (80.5457, 78.8085) (80.873, 78.8085) (81.2339, 79.1213) (81.2339, 79.3234) knots 0 0 0 1 2 2 2
  spline S21 degree 2 poles (81.2339, 79.3234) (81.2339, 79.5159) (81.0606, 79.6699) knots 0 0 0 1 1 1
  spline S22 degree 2 poles (81.0606, 79.6699) (80.8922, 79.8239) (80.2714, 79.9634) knots 0 0 0 1 1 1
  spline S23 degree 2 poles (80.2714, 79.9634) (79.2512, 80.1896) (78.8181, 80.5698) knots 0 0 0 1 1 1
  spline S24 degree 2 poles (78.8181, 80.5698) (78.3802, 80.95) (78.3802, 81.5371) knots 0 0 0 1 1 1
  spline S25 degree 2 poles (78.3802, 81.5371) (78.3802, 81.922) (78.8277, 82.6054) (79.7276, 83) (80.5072, 83) knots 0 0 0 1 2 3 3 3
  spline S26 degree 2 poles (80.5072, 83) (81.4697, 83) (82.4755, 82.2878) (82.5717, 81.5082) knots 0 0 0 1 2 2 2
  line L54 (82.5717, 81.5082) -> (81.1136, 81.4216)
  spline S27 degree 2 poles (81.1136, 81.4216) (81.0558, 81.7584) (80.6805, 82.0664) (80.3532, 82.0664) knots 0 0 0 1 2 2 2
  spline S28 degree 2 poles (80.3532, 82.0664) (80.0837, 82.0664) (79.8094, 81.8402) (79.8094, 81.6718) knots 0 0 0 1 2 2 2
  spline S29 degree 2 poles (79.8094, 81.6718) (79.8094, 81.5563) (79.9249, 81.4601) knots 0 0 0 1 1 1
  spline S30 degree 2 poles (79.9249, 81.4601) (80.0356, 81.359) (80.4447, 81.2772) knots 0 0 0 1 1 1
  spline S31 degree 2 poles (80.4447, 81.2772) (81.4601, 81.0558) (82.3359, 80.6083) (82.7353, 79.949) (82.7353, 79.5399) knots 0 0 0 1 2 3 3 3
  spline S32 degree 2 poles (82.7353, 79.5399) (82.7353, 79.0587) (82.2012, 78.2454) (81.2483, 77.8268) (80.5168, 77.8268) knots 0 0 0 1 2 3 3 3
  spline S33 degree 2 poles (80.5168, 77.8268) (79.2416, 77.8268) (78.2551, 78.8085) (78.1925, 79.5688) knots 0 0 0 1 2 2 2
  line L55 (51.2772, 71.8964) -> (52.8219, 71.8964)
  line L56 (52.8219, 71.8964) -> (52.8219, 68.1284)
  line L57 (52.8219, 68.1284) -> (55.2329, 68.1284)
  line L58 (55.2329, 68.1284) -> (55.2329, 66.8964)
  line L59 (55.2329, 66.8964) -> (51.2772, 66.8964)
  line L60 (51.2772, 66.8964) -> (51.2772, 71.8964)
  line L61 (56.0029, 71.8964) -> (57.5525, 71.8964)
  line L62 (57.5525, 71.8964) -> (57.5525, 66.8964)
  line L63 (57.5525, 66.8964) -> (56.0029, 66.8964)
  line L64 (56.0029, 66.8964) -> (56.0029, 71.8964)
  spline S34 degree 2 poles (63.1059, 67.6231) (63.3946, 67.421) (63.4812, 67.3728) knots 0 0 0 1 1 1
  spline S35 degree 2 poles (63.4812, 67.3728) (63.616, 67.2958) (63.8422, 67.1996) knots 0 0 0 1 1 1
  line L65 (63.8422, 67.1996) -> (63.409, 66.3334)
  spline S36 degree 2 poles (63.409, 66.3334) (63.0866, 66.4922) (62.4514, 66.9205) (62.3263, 67.0312) knots 0 0 0 1 2 2 2
  spline S37 degree 2 poles (62.3263, 67.0312) (61.8162, 66.8098) (61.0414, 66.8098) knots 0 0 0 1 1 1
  spline S38 degree 2 poles (61.0414, 66.8098) (59.9057, 66.8098) (59.2464, 67.4017) knots 0 0 0 1 1 1
  spline S39 degree 2 poles (59.2464, 67.4017) (58.4668, 68.1043) (58.4668, 69.3796) knots 0 0 0 1 1 1
  spline S40 degree 2 poles (58.4668, 69.3796) (58.4668, 70.6163) (59.8287, 71.983) (61.051, 71.983) knots 0 0 0 1 2 2 2
  spline S41 degree 2 poles (61.051, 71.983) (62.2974, 71.983) (63.6497, 70.6452) (63.6497, 69.3988) knots 0 0 0 1 2 2 2
  spline S42 degree 2 poles (63.6497, 69.3988) (63.6497, 68.292) (63.1059, 67.6231) knots 0 0 0 1 1 1
  spline S43 degree 2 poles (61.922, 68.4171) (62.1049, 68.7492) (62.1049, 69.4084) knots 0 0 0 1 1 1
  spline S44 degree 2 poles (62.1049, 69.4084) (62.1049, 70.164) (61.5419, 70.8136) (61.0462, 70.8136) knots 0 0 0 1 2 2 2
  spline S45 degree 2 poles (61.0462, 70.8136) (60.5842, 70.8136) (60.0115, 70.1495) (60.0115, 69.4469) knots 0 0 0 1 2 2 2
  spline S46 degree 2 poles (60.0115, 69.4469) (60.0115, 68.6288) (60.5698, 67.9647) (61.0606, 67.9647) knots 0 0 0 1 2 2 2
  spline S47 degree 2 poles (61.0606, 67.9647) (61.2146, 67.9647) (61.3542, 67.9936) knots 0 0 0 1 1 1
  spline S48 degree 2 poles (61.3542, 67.9936) (61.1617, 68.1813) (60.743, 68.3497) knots 0 0 0 1 1 1
  line L66 (60.743, 68.3497) -> (60.9836, 68.908)
  spline S49 degree 2 poles (60.9836, 68.908) (61.1906, 68.8695) (61.4167, 68.7588) (61.7488, 68.5278) knots 0 0 0 1 2 2 2
  spline S50 degree 2 poles (61.7488, 68.5278) (61.8258, 68.4749) (61.922, 68.4171) knots 0 0 0 1 1 1
  line L67 (67.7449, 71.8964) -> (69.2849, 71.8964)
  line L68 (69.2849, 71.8964) -> (69.2849, 68.9176)
  spline S51 degree 2 poles (69.2849, 68.9176) (69.2849, 68.4749) (69.0106, 67.6856) (68.4187, 67.0985) (68.0914, 66.9782) knots 0 0 0 1 2 3 3 3
  spline S52 degree 2 poles (68.0914, 66.9782) (67.6439, 66.8098) (67.0087, 66.8098) knots 0 0 0 1 1 1
  spline S53 degree 2 poles (67.0087, 66.8098) (66.6429, 66.8098) (65.7815, 66.9108) (65.1992, 67.214) (64.718, 67.7723) (64.6314, 68.0706) knots 0 0 0 1 2 3 4 4 4
  spline S54 degree 2 poles (64.6314, 68.0706) (64.487, 68.547) (64.487, 68.9176) knots 0 0 0 1 1 1
  line L69 (64.487, 68.9176) -> (64.487, 71.8964)
  line L70 (64.487, 71.8964) -> (66.0269, 71.8964)
  line L71 (66.0269, 71.8964) -> (66.0269, 68.8454)
  spline S55 degree 2 poles (66.0269, 68.8454) (66.0269, 68.4364) (66.4841, 67.9744) (66.8884, 67.9744) knots 0 0 0 1 2 2 2
  spline S56 degree 2 poles (66.8884, 67.9744) (67.2878, 67.9744) (67.7449, 68.4267) (67.7449, 68.8454) knots 0 0 0 1 2 2 2
  line L72 (67.7449, 68.8454) -> (67.7449, 71.8964)
  line L73 (70.3677, 71.8964) -> (71.9172, 71.8964)
  line L74 (71.9172, 71.8964) -> (71.9172, 66.8964)
  line L75 (71.9172, 66.8964) -> (70.3677, 66.8964)
  line L76 (70.3677, 66.8964) -> (70.3677, 71.8964)
  line L77 (73.0481, 71.8964) -> (75.3436, 71.8964)
  spline S57 degree 2 poles (75.3436, 71.8964) (76.0221, 71.8964) (76.8595, 71.5259) (77.4033, 70.8377) (77.6487, 69.9234) (77.6487, 69.4133) knots 0 0 0 1 2 3 4 4 4
  spline S58 degree 2 poles (77.6487, 69.4133) (77.6487, 68.6096) (77.283, 67.7289) (76.6381, 67.1322) (76.2628, 67.0312) knots 0 0 0 1 2 3 3 3
  spline S59 degree 2 poles (76.2628, 67.0312) (75.7575, 66.8964) (75.3436, 66.8964) knots 0 0 0 1 1 1
  line L78 (75.3436, 66.8964) -> (73.0481, 66.8964)
  line L79 (73.0481, 66.8964) -> (73.0481, 71.8964)
  line L80 (74.5929, 70.7655) -> (74.5929, 68.0321)
  line L81 (74.5929, 68.0321) -> (74.9731, 68.0321)
  spline S60 degree 2 poles (74.9731, 68.0321) (75.4543, 68.0321) (75.8633, 68.2487) (76.0943, 68.7828) (76.0943, 69.3844) knots 0 0 0 1 2 3 3 3
  spline S61 degree 2 poles (76.0943, 69.3844) (76.0943, 70.1784) (75.5746, 70.7655) (74.9779, 70.7655) knots 0 0 0 1 2 2 2
  line L82 (74.9779, 70.7655) -> (74.5929, 70.7655)
  line L83 (78.1925, 68.5519) -> (79.6651, 68.6433)
  spline S62 degree 2 poles (79.6651, 68.6433) (79.7132, 68.2824) (79.8576, 68.0947) knots 0 0 0 1 1 1
  spline S63 degree 2 poles (79.8576, 68.0947) (80.0982, 67.7915) (80.5457, 67.7915) knots 0 0 0 1 1 1
  spline S64 degree 2 poles (80.5457, 67.7915) (80.873, 67.7915) (81.2339, 68.1043) (81.2339, 68.3064) knots 0 0 0 1 2 2 2
  spline S65 degree 2 poles (81.2339, 68.3064) (81.2339, 68.4989) (81.0606, 68.6529) knots 0 0 0 1 1 1
  spline S66 degree 2 poles (81.0606, 68.6529) (80.8922, 68.8069) (80.2714, 68.9465) knots 0 0 0 1 1 1
  spline S67 degree 2 poles (80.2714, 68.9465) (79.2512, 69.1726) (78.8181, 69.5528) knots 0 0 0 1 1 1
  spline S68 degree 2 poles (78.8181, 69.5528) (78.3802, 69.933) (78.3802, 70.5201) knots 0 0 0 1 1 1
  spline S69 degree 2 poles (78.3802, 70.5201) (78.3802, 70.9051) (78.8277, 71.5884) (79.7276, 71.983) (80.5072, 71.983) knots 0 0 0 1 2 3 3 3
  spline S70 degree 2 poles (80.5072, 71.983) (81.4697, 71.983) (82.4755, 71.2708) (82.5717, 70.4912) knots 0 0 0 1 2 2 2
  line L84 (82.5717, 70.4912) -> (81.1136, 70.4046)
  spline S71 degree 2 poles (81.1136, 70.4046) (81.0558, 70.7415) (80.6805, 71.0494) (80.3532, 71.0494) knots 0 0 0 1 2 2 2
  spline S72 degree 2 poles (80.3532, 71.0494) (80.0837, 71.0494) (79.8094, 70.8233) (79.8094, 70.6548) knots 0 0 0 1 2 2 2
  spline S73 degree 2 poles (79.8094, 70.6548) (79.8094, 70.5393) (79.9249, 70.4431) knots 0 0 0 1 1 1
  spline S74 degree 2 poles (79.9249, 70.4431) (80.0356, 70.342) (80.4447, 70.2602) knots 0 0 0 1 1 1
  spline S75 degree 2 poles (80.4447, 70.2602) (81.4601, 70.0389) (82.3359, 69.5913) (82.7353, 68.932) (82.7353, 68.523) knots 0 0 0 1 2 3 3 3
  spline S76 degree 2 poles (82.7353, 68.523) (82.7353, 68.0417) (82.2012, 67.2285) (81.2483, 66.8098) (80.5168, 66.8098) knots 0 0 0 1 2 3 3 3
  spline S77 degree 2 poles (80.5168, 66.8098) (79.2416, 66.8098) (78.2551, 67.7915) (78.1925, 68.5519) knots 0 0 0 1 2 2 2
  line L85 (-82.4803, 82.9134) -> (-78.6641, 82.9134)
  line L86 (-78.6641, 82.9134) -> (-78.6641, 81.8402)
  line L87 (-78.6641, 81.8402) -> (-80.9259, 81.8402)
  line L88 (-80.9259, 81.8402) -> (-80.9259, 80.9692)
  line L89 (-80.9259, 80.9692) -> (-78.9962, 80.9692)
  line L90 (-78.9962, 80.9692) -> (-78.9962, 79.9586)
  line L91 (-78.9962, 79.9586) -> (-80.9259, 79.9586)
  line L92 (-80.9259, 79.9586) -> (-80.9259, 77.9134)
  line L93 (-80.9259, 77.9134) -> (-82.4803, 77.9134)
  line L94 (-82.4803, 77.9134) -> (-82.4803, 82.9134)
  line L95 (-77.8027, 77.9134) -> (-77.8027, 82.9134)
  line L96 (-77.8027, 82.9134) -> (-75.2281, 82.9134)
  spline S78 degree 2 poles (-75.2281, 82.9134) (-74.5159, 82.9134) (-73.7555, 82.668) (-73.2936, 82.0038) (-73.2936, 81.5274) knots 0 0 0 1 2 3 3 3
  spline S79 degree 2 poles (-73.2936, 81.5274) (-73.2936, 81.1088) (-73.6497, 80.5072) (-73.9577, 80.3195) knots 0 0 0 1 2 2 2
  spline S80 degree 2 poles (-73.9577, 80.3195) (-74.155, 80.1992) (-74.5014, 80.1222) knots 0 0 0 1 1 1
  spline S81 degree 2 poles (-74.5014, 80.1222) (-74.2271, 80.0308) (-74.0972, 79.9394) knots 0 0 0 1 1 1
  spline S82 degree 2 poles (-74.0972, 79.9394) (-74.0154, 79.8768) (-73.693, 79.4726) (-73.6352, 79.3619) knots 0 0 0 1 2 2 2
  line L97 (-73.6352, 79.3619) -> (-72.8893, 77.9134)
  line L98 (-72.8893, 77.9134) -> (-74.6362, 77.9134)
  line L99 (-74.6362, 77.9134) -> (-75.4591, 79.4437)
  spline S83 degree 2 poles (-75.4591, 79.4437) (-75.6131, 79.7372) (-75.7334, 79.8287) knots 0 0 0 1 1 1
  spline S84 degree 2 poles (-75.7334, 79.8287) (-75.9018, 79.9442) (-76.1136, 79.9442) knots 0 0 0 1 1 1
  line L100 (-76.1136, 79.9442) -> (-76.2483, 79.9442)
  line L101 (-76.2483, 79.9442) -> (-76.2483, 77.9134)
  line L102 (-76.2483, 77.9134) -> (-77.8027, 77.9134)
  line L103 (-76.2483, 80.8874) -> (-75.5987, 80.8874)
  spline S85 degree 2 poles (-75.5987, 80.8874) (-75.4976, 80.8874) (-75.1944, 80.9548) knots 0 0 0 1 1 1
  spline S86 degree 2 poles (-75.1944, 80.9548) (-75.0404, 80.9885) (-74.8479, 81.2387) (-74.8479, 81.4023) knots 0 0 0 1 2 2 2
  spline S87 degree 2 poles (-74.8479, 81.4023) (-74.8479, 81.6429) (-75.1511, 81.9028) (-75.5746, 81.9028) knots 0 0 0 1 2 2 2
  line L104 (-75.5746, 81.9028) -> (-76.2483, 81.9028)
  line L105 (-76.2483, 81.9028) -> (-76.2483, 80.8874)
  line L106 (-69.3138, 78.7411) -> (-71.0703, 78.7411)
  line L107 (-71.0703, 78.7411) -> (-71.3157, 77.9134)
  line L108 (-71.3157, 77.9134) -> (-72.8941, 77.9134)
  line L109 (-72.8941, 77.9134) -> (-71.0125, 82.9134)
  line L110 (-71.0125, 82.9134) -> (-69.3234, 82.9134)
  line L111 (-69.3234, 82.9134) -> (-67.4466, 77.9134)
  line L112 (-67.4466, 77.9134) -> (-69.0635, 77.9134)
  line L113 (-69.0635, 77.9134) -> (-69.3138, 78.7411)
  line L114 (-69.6362, 79.8239) -> (-70.1848, 81.6189)
  line L115 (-70.1848, 81.6189) -> (-70.7334, 79.8239)
  line L116 (-70.7334, 79.8239) -> (-69.6362, 79.8239)
  line L117 (-64.4293, 79.7228) -> (-64.4293, 80.7623)
  line L118 (-64.4293, 80.7623) -> (-62.0423, 80.7623)
  line L119 (-62.0423, 80.7623) -> (-62.0423, 78.6352)
  spline S88 degree 2 poles (-62.0423, 78.6352) (-62.7305, 78.1636) (-63.7844, 77.8268) (-64.5063, 77.8268) knots 0 0 0 1 2 2 2
  spline S89 degree 2 poles (-64.5063, 77.8268) (-65.3965, 77.8268) (-66.5226, 78.4331) (-67.1386, 79.6362) (-67.1386, 80.4158) knots 0 0 0 1 2 3 3 3
  spline S90 degree 2 poles (-67.1386, 80.4158) (-67.1386, 81.2339) (-66.4649, 82.4418) (-65.8104, 82.7594) knots 0 0 0 1 2 2 2
  spline S91 degree 2 poles (-65.8104, 82.7594) (-65.3003, 83) (-64.4437, 83) knots 0 0 0 1 1 1
  spline S92 degree 2 poles (-64.4437, 83) (-63.6112, 83) (-62.7883, 82.7016) (-62.2445, 82.0664) (-62.1097, 81.5852) knots 0 0 0 1 2 3 3 3
  line L120 (-62.1097, 81.5852) -> (-63.6015, 81.3157)
  spline S93 degree 2 poles (-63.6015, 81.3157) (-63.693, 81.5996) (-64.1357, 81.9028) (-64.4774, 81.9028) knots 0 0 0 1 2 2 2
  spline S94 degree 2 poles (-64.4774, 81.9028) (-64.9827, 81.9028) (-65.589, 81.1954) (-65.589, 80.4302) knots 0 0 0 1 2 2 2
  spline S95 degree 2 poles (-65.589, 80.4302) (-65.589, 79.6218) (-64.9779, 78.924) (-64.4293, 78.924) knots 0 0 0 1 2 2 2
  spline S96 degree 2 poles (-64.4293, 78.924) (-64.1694, 78.924) (-63.6978, 79.0731) (-63.3946, 79.256) knots 0 0 0 1 2 2 2
  line L121 (-63.3946, 79.256) -> (-63.3946, 79.7228)
  line L122 (-63.3946, 79.7228) -> (-64.4293, 79.7228)
  line L123 (-61.0654, 82.9134) -> (-59.5159, 82.9134)
  line L124 (-59.5159, 82.9134) -> (-59.5159, 77.9134)
  line L125 (-59.5159, 77.9134) -> (-61.0654, 77.9134)
  line L126 (-61.0654, 77.9134) -> (-61.0654, 82.9134)
  line L127 (-58.409, 82.9134) -> (-56.8643, 82.9134)
  line L128 (-56.8643, 82.9134) -> (-56.8643, 79.1453)
  line L129 (-56.8643, 79.1453) -> (-54.4533, 79.1453)
  line L130 (-54.4533, 79.1453) -> (-54.4533, 77.9134)
  line L131 (-54.4533, 77.9134) -> (-58.409, 77.9134)
  line L132 (-58.409, 77.9134) -> (-58.409, 82.9134)
  line L133 (-53.7459, 82.9134) -> (-49.6073, 82.9134)
  line L134 (-49.6073, 82.9134) -> (-49.6073, 81.845)
  line L135 (-49.6073, 81.845) -> (-52.1963, 81.845)
  line L136 (-52.1963, 81.845) -> (-52.1963, 81.051)
  line L137 (-52.1963, 81.051) -> (-49.795, 81.051)
  line L138 (-49.795, 81.051) -> (-49.795, 80.0308)
  line L139 (-49.795, 80.0308) -> (-52.1963, 80.0308)
  line L140 (-52.1963, 80.0308) -> (-52.1963, 79.0443)
  line L141 (-52.1963, 79.0443) -> (-49.5303, 79.0443)
  line L142 (-49.5303, 79.0443) -> (-49.5303, 77.9134)
  line L143 (-49.5303, 77.9134) -> (-53.7459, 77.9134)
  line L144 (-53.7459, 77.9134) -> (-53.7459, 82.9134)
  line L145 (-79.9682, 68.7058) -> (-79.9682, 69.7453)
  line L146 (-79.9682, 69.7453) -> (-77.5813, 69.7453)
  line L147 (-77.5813, 69.7453) -> (-77.5813, 67.6183)
  spline S97 degree 2 poles (-77.5813, 67.6183) (-78.2695, 67.1467) (-79.3234, 66.8098) (-80.0452, 66.8098) knots 0 0 0 1 2 2 2
  spline S98 degree 2 poles (-80.0452, 66.8098) (-80.9355, 66.8098) (-82.0616, 67.4161) (-82.6776, 68.6192) (-82.6776, 69.3988) knots 0 0 0 1 2 3 3 3
  spline S99 degree 2 poles (-82.6776, 69.3988) (-82.6776, 70.2169) (-82.0038, 71.4248) (-81.3494, 71.7424) knots 0 0 0 1 2 2 2
  spline S100 degree 2 poles (-81.3494, 71.7424) (-80.8393, 71.983) (-79.9827, 71.983) knots 0 0 0 1 1 1
  spline S101 degree 2 poles (-79.9827, 71.983) (-79.1501, 71.983) (-78.3272, 71.6847) (-77.7834, 71.0494) (-77.6487, 70.5682) knots 0 0 0 1 2 3 3 3
  line L148 (-77.6487, 70.5682) -> (-79.1405, 70.2987)
  spline S102 degree 2 poles (-79.1405, 70.2987) (-79.232, 70.5826) (-79.6747, 70.8858) (-80.0164, 70.8858) knots 0 0 0 1 2 2 2
  spline S103 degree 2 poles (-80.0164, 70.8858) (-80.5217, 70.8858) (-81.128, 70.1784) (-81.128, 69.4133) knots 0 0 0 1 2 2 2
  spline S104 degree 2 poles (-81.128, 69.4133) (-81.128, 68.6048) (-80.5168, 67.907) (-79.9682, 67.907) knots 0 0 0 1 2 2 2
  spline S105 degree 2 poles (-79.9682, 67.907) (-79.7084, 67.907) (-79.2368, 68.0562) (-78.9336, 68.239) knots 0 0 0 1 2 2 2
  line L149 (-78.9336, 68.239) -> (-78.9336, 68.7058)
  line L150 (-78.9336, 68.7058) -> (-79.9682, 68.7058)
  line L151 (-76.667, 71.8964) -> (-75.1222, 71.8964)
  line L152 (-75.1222, 71.8964) -> (-75.1222, 68.1284)
  line L153 (-75.1222, 68.1284) -> (-72.7113, 68.1284)
  line L154 (-72.7113, 68.1284) -> (-72.7113, 66.8964)
  line L155 (-72.7113, 66.8964) -> (-76.667, 66.8964)
  line L156 (-76.667, 66.8964) -> (-76.667, 71.8964)
  line L157 (-68.9288, 67.7241) -> (-70.6853, 67.7241)
  line L158 (-70.6853, 67.7241) -> (-70.9307, 66.8964)
  line L159 (-70.9307, 66.8964) -> (-72.5091, 66.8964)
  line L160 (-72.5091, 66.8964) -> (-70.6275, 71.8964)
  line L161 (-70.6275, 71.8964) -> (-68.9384, 71.8964)
  line L162 (-68.9384, 71.8964) -> (-67.0616, 66.8964)
  line L163 (-67.0616, 66.8964) -> (-68.6785, 66.8964)
  line L164 (-68.6785, 66.8964) -> (-68.9288, 67.7241)
  line L165 (-69.2512, 68.8069) -> (-69.7998, 70.6019)
  line L166 (-69.7998, 70.6019) -> (-70.3484, 68.8069)
  line L167 (-70.3484, 68.8069) -> (-69.2512, 68.8069)
  line L168 (-66.8354, 68.5519) -> (-65.3628, 68.6433)
  spline S106 degree 2 poles (-65.3628, 68.6433) (-65.3147, 68.2824) (-65.1704, 68.0947) knots 0 0 0 1 1 1
  spline S107 degree 2 poles (-65.1704, 68.0947) (-64.9297, 67.7915) (-64.4822, 67.7915) knots 0 0 0 1 1 1
  spline S108 degree 2 poles (-64.4822, 67.7915) (-64.155, 67.7915) (-63.794, 68.1043) (-63.794, 68.3064) knots 0 0 0 1 2 2 2
  spline S109 degree 2 poles (-63.794, 68.3064) (-63.794, 68.4989) (-63.9673, 68.6529) knots 0 0 0 1 1 1
  spline S110 degree 2 poles (-63.9673, 68.6529) (-64.1357, 68.8069) (-64.7565, 68.9465) knots 0 0 0 1 1 1
  spline S111 degree 2 poles (-64.7565, 68.9465) (-65.7767, 69.1726) (-66.2098, 69.5528) knots 0 0 0 1 1 1
  spline S112 degree 2 poles (-66.2098, 69.5528) (-66.6477, 69.933) (-66.6477, 70.5201) knots 0 0 0 1 1 1
  spline S113 degree 2 poles (-66.6477, 70.5201) (-66.6477, 70.9051) (-66.2002, 71.5884) (-65.3003, 71.983) (-64.5207, 71.983) knots 0 0 0 1 2 3 3 3
  spline S114 degree 2 poles (-64.5207, 71.983) (-63.5582, 71.983) (-62.5525, 71.2708) (-62.4562, 70.4912) knots 0 0 0 1 2 2 2
  line L169 (-62.4562, 70.4912) -> (-63.9143, 70.4046)
  spline S115 degree 2 poles (-63.9143, 70.4046) (-63.9721, 70.7415) (-64.3474, 71.0494) (-64.6747, 71.0494) knots 0 0 0 1 2 2 2
  spline S116 degree 2 poles (-64.6747, 71.0494) (-64.9442, 71.0494) (-65.2185, 70.8233) (-65.2185, 70.6548) knots 0 0 0 1 2 2 2
  spline S117 degree 2 poles (-65.2185, 70.6548) (-65.2185, 70.5393) (-65.103, 70.4431) knots 0 0 0 1 1 1
  spline S118 degree 2 poles (-65.103, 70.4431) (-64.9923, 70.342) (-64.5833, 70.2602) knots 0 0 0 1 1 1
  spline S119 degree 2 poles (-64.5833, 70.2602) (-63.5679, 70.0389) (-62.692, 69.5913) (-62.2926, 68.932) (-62.2926, 68.523) knots 0 0 0 1 2 3 3 3